makerbeam-10mm-corner-no-support v2 (Autodesk Fusion 360 design; units mm, degrees)
Autodesk Fusion 360 part; units mm, degrees
box "BoxPrimitive1" add length 35 width 12 height 12 placed x (0, 0, -1) y (-1, 0, 0) z (0, 1, 0) at (12, 0, 0)
box "BoxPrimitive2" add length 12 width 35 height 12 placed x (0, 0, -1) y (-1, 0, 0) z (0, 1, 0) at (35, 0, 0)
box "BoxPrimitive3" add length 12 width 12 height 35 placed x (0, 0, -1) y (-1, 0, 0) z (0, 1, 0) at (12, 0, 0)
cylinder "CylinderPrimitive1" cut diameter 3 height 15 placed x (1, 0, 0) y (0, 0, -1) z (0, 1, 0) at (30, 0, -5)
cylinder "CylinderPrimitive2" cut diameter 3 height 15 placed x (1, 0, 0) y (0, 0, -1) z (0, 1, 0) at (20, 0, -5)
cylinder "CylinderPrimitive3" cut diameter 3 height 15 placed x (1, 0, 0) y (0, 0, -1) z (0, 1, 0) at (5, 0, -30)
cylinder "CylinderPrimitive4" cut diameter 3 height 15 placed x (1, 0, 0) y (0, 0, -1) z (0, 1, 0) at (5, 0, -20)
cylinder "CylinderPrimitive5" cut diameter 3 height 15 placed x (0, 0, -1) y (0, 1, 0) z (1, 0, 0) at (0, 5, -30)
cylinder "CylinderPrimitive6" cut diameter 3 height 15 placed x (0, 0, -1) y (0, 1, 0) z (1, 0, 0) at (0, 5, -20)
cylinder "CylinderPrimitive7" cut diameter 3 height -15 placed x (0, 1, 0) y (1, 0, 0) z (0, 0, -1) at (30, 5, -12)
cylinder "CylinderPrimitive8" cut diameter 3 height -15 placed x (0, 1, 0) y (1, 0, 0) z (0, 0, -1) at (20, 5, -12)
cylinder "CylinderPrimitive9" cut diameter 3 height -15 placed x (0, 0, -1) y (0, 1, 0) z (1, 0, 0) at (12, 30, -5)
cylinder "CylinderPrimitive10" cut diameter 3 height -15 placed x (0, 0, -1) y (0, 1, 0) z (1, 0, 0) at (12, 20, -5)
cylinder "CylinderPrimitive11" cut diameter 3 height -15 placed x (0, 1, 0) y (1, 0, 0) z (0, 0, -1) at (5, 30, -12)
cylinder "CylinderPrimitive12" cut diameter 3 height -15 placed x (0, 1, 0) y (1, 0, 0) z (0, 0, -1) at (5, 20, -12)
box "BoxPrimitive7" cut length 45 width 50 height 10 placed x (0, 0, -1) y (-1, 0, 0) z (0, 1, 0) at (40, 0, 0)
box "BoxPrimitive9" cut length 52 width 10 height -10 placed x (0, 1, 0) y (-1, 0, 0) z (0, 0, 1) at (10, -12, 0)
sketch "Sketch32" plane through (0, 0, -12) normal (0, 0, -1) x (-1, 0, 0)
  circle A0 centre (-5, 20) radius 1.5
  circle A1 centre (-5, 30) radius 1.5
  line L0 (-12, 12) -> (0, 12)
  line L1 (0, 12) -> (0, 35)
  line L2 (0, 35) -> (-12, 35)
  line L3 (-12, 35) -> (-12, 12)
  line L4 (-12, 35) -> (-35, 12)
  line L5 (-35, 12) -> (-12, 12)
  point P0 (-35, 12)
extrude "Extrude8" add sketch "Sketch32" against normal blind 2 contours L3 L4 L5
sketch "Sketch33" plane through (12, 0, 0) normal (1, 0, 0) x (0, 0, -1)
  line L0 (10, 12) -> (10, 35)
  line L1 (10, 35) -> (0, 35)
  line L2 (0, 35) -> (0, 12)
  line L3 (0, 12) -> (10, 12)
  circle A0 centre (5, 30) radius 1.5
  circle A1 centre (5, 20) radius 1.5
  line L4 (12, 35) -> (35, 12)
  line L5 (35, 12) -> (12, 12)
  line L6 (12, 12) -> (12, 35)
  point P0 (12, 35)
  point P1 (35, 12)
  point P2 (12, 12)
extrude "Extrude9" add sketch "Sketch33" against normal blind 2 contours L4 L5 L6
sketch "Sketch34" plane through (0, 12, 0) normal (0, 1, 0) x (-1, 0, 0)
  line L0 (-35, -10) -> (-12, -10)
  line L1 (-12, -10) -> (-12, 0)
  line L2 (-12, 0) -> (-35, 0)
  line L3 (-35, 0) -> (-35, -10)
  circle A0 centre (-30, -5) radius 1.5
  circle A1 centre (-20, -5) radius 1.5
  line L4 (-12, -35) -> (-35, -12)
  line L5 (-35, -12) -> (-12, -12)
  line L6 (-12, -12) -> (-12, -35)
  point P0 (-12, -35)
  point P1 (-35, -12)
  point P2 (-12, -12)
  point P3 (-12, -35)
extrude "Extrude10" add sketch "Sketch34" against normal blind 2 contours L4 L5 L6
cylinder "CylinderPrimitive13" cut diameter 3 height 15 placed x (1, 0, 0) y (0, 0, -1) z (0, 1, 0) at (20, 0, -20)
cylinder "CylinderPrimitive14" cut diameter 3 height -15 placed x (0, 0, -1) y (0, 1, 0) z (1, 0, 0) at (12, 20, -20)
cylinder "CylinderPrimitive15" cut diameter 3 height -15 placed x (0, 1, 0) y (1, 0, 0) z (0, 0, -1) at (20, 20, -12)
